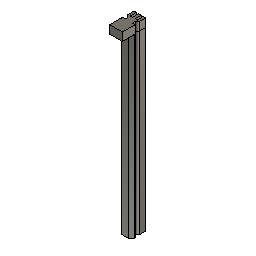
Car Front Cover Slider v1 (Autodesk Fusion 360 design; units mm, degrees)
Autodesk Fusion 360 part; units mm, degrees
note: some values were not read from the file. Set by a fixed rule: which sketch regions a step uses.
sketch "Sketch1" plane through (0, 0, 0) normal (0, 0, 1) x (1, 0, 0)
  line L0 (6.9, 0.5) -> (6.9, -1.8)
  line L1 (6.9, -1.8) -> (4.6, -1.8)
  line L2 (4.6, -1.8) -> (4.6, -2.8)
  line L3 (4.6, -2.8) -> (6.9335, -5.1335)
  line L4 (4.6, -2.8) -> (7.9, -2.8) construction
  line L5 (4.6, -1.8) -> (10.8, -1.8)
  line L6 (6.9, -1.8) -> (13.1, -1.8)
  line L7 (13.1, -1.8) -> (15.4273, -1.8)
  line L8 (15.4273, -1.8) -> (15.4273, -2.8)
  line L9 (15.4273, -2.8) -> (13.0938, -5.1335)
  line L10 (13.0938, -5.1335) -> (6.9335, -5.1335)
  line L11 (15.4273, -1.8) -> (13.1, -1.8)
  line L12 (13.1, -1.8) -> (13.1, 0.5)
  line L13 (6.9, 0.5) -> (4.9, 0.5)
  line L14 (4.9, 0.5) -> (4.9, 7.6)
  line L15 (4.9, 7.6) -> (6.9, 7.6)
  line L16 (6.9, 7.6) -> (6.9, 2.5)
  line L17 (6.9, 2.5) -> (8.875, 2.5)
  line L18 (8.875, 2.5) -> (8.875, 7.6)
  line L19 (8.875, 7.6) -> (10.925, 7.6)
  line L20 (10.925, 7.6) -> (10.925, 2.5)
  line L21 (10.925, 2.5) -> (12.9, 2.5)
  line L22 (12.9, 2.5) -> (12.9, 7.6)
  line L23 (12.9, 7.6) -> (14.9, 7.6)
  line L24 (14.9, 7.6) -> (14.9, 0.5)
  line L25 (14.9, 0.5) -> (13.1, 0.5)
  dimension "d2" = 2.3
  dimension "d3" = 2.3
  dimension "d4" = 1
  dimension "d5" = 45
  dimension "d6" = 3.3
  dimension "d7" = 6.2
  dimension "d11" = 6.2
  dimension "d12" = 135
  dimension "d13" = 3.3
  dimension "d127" = 2.3
  dimension "d128" = 2
  dimension "d129" = 7.1
  dimension "d130" = 2
  dimension "d131" = 5.1
  dimension "d132" = 1.975
  dimension "d133" = 2.05
  dimension "d134" = 1.975
  dimension "d135" = 2
  dimension "d136" = 7.1
  dimension "d143" = 2
  dimension "d144" = 5.1
  constraint perpendicular L0 L1
  constraint perpendicular L1 L2
  constraint horizontal L4
  constraint perpendicular L2 L5
  constraint perpendicular L0 L6
  constraint parallel L6 L7
  constraint perpendicular L7 L8
  constraint perpendicular L11 L12
  constraint perpendicular L0 L13
  constraint perpendicular L13 L14
  constraint perpendicular L14 L15
  constraint perpendicular L15 L16
  constraint perpendicular L16 L17
  constraint perpendicular L17 L18
  constraint perpendicular L18 L19
  constraint perpendicular L19 L20
  constraint perpendicular L20 L21
  constraint perpendicular L21 L22
  constraint perpendicular L22 L23
  constraint perpendicular L21 L24
  constraint perpendicular L12 L25
  measures "d2" distance of L0.start L0.end
  measures "d3" distance of L0.end L1.end
  measures "d4" distance of L1.end L2.end
  measures "d5" angle of L3 L4
  measures "d6" distance of L2.end L3.end
  measures "d7" distance of L1.end L5.end
  measures "d11" distance of L0.end L6.end
  measures "d12" angle of L8 L9
  measures "d13" distance of L8.end L9.end
  measures "d127" distance of L6.end L12.end
  measures "d128" distance of L0.start L13.end
  measures "d129" distance of L13.end L14.end
  measures "d130" distance of L14.end L15.end
  measures "d131" distance of L15.end L16.end
  measures "d132" distance of L16.end L17.end
  measures "d133" distance of L18.end L19.end
  measures "d134" distance of L20.end L21.end
  measures "d135" distance of L22.end L23.end
  measures "d136" distance of L23.end L24.end
  measures "d143" distance of L21 L25
  measures "d144" distance of L19.end L20.end
extrude "Extrude1" add sketch "Sketch1" along normal blind 150 makes body 1
fillet "Fillet5" radius 2 2 edges at (14.9, 0.5, 75) (4.9, 0.5, 75) on bodies 1
sketch "Sketch12" plane through (0, 0, 150) normal (0, 0, 1) x (-1, 0, 0)
  arc A0 (-4.9, -2.5) -> (-6.9, -0.5) centre (-6.9, -2.5) ccw
  line L0 (-6.9, -0.5) -> (-6.9, 1.8)
  line L1 (-6.9, 1.8) -> (-4.6, 1.8)
  line L2 (-4.6, 1.8) -> (-4.6, 2.8)
  line L3 (-4.6, 2.8) -> (-6.9335, 5.1335)
  line L4 (-6.9335, 5.1335) -> (-13.0938, 5.1335)
  line L5 (-13.0938, 5.1335) -> (-15.4273, 2.8)
  line L6 (-15.4273, 2.8) -> (-15.4273, 1.8)
  line L7 (-15.4273, 1.8) -> (-13.1, 1.8)
  line L8 (-13.1, 1.8) -> (-13.1, -0.5)
  arc A1 (-13.1, -0.5) -> (-14.9, -2.49) centre (-12.9, -2.49) ccw
  line L9 (-14.9, -2.49) -> (-14.9, -7.6)
  line L10 (-14.9, -7.6) -> (-12.9, -7.6)
  line L11 (-12.9, -7.6) -> (-12.9, -2.5)
  line L12 (-12.9, -2.5) -> (-10.925, -2.5)
  line L13 (-10.925, -2.5) -> (-10.925, -7.6)
  line L14 (-10.925, -7.6) -> (-8.875, -7.6)
  line L15 (-8.875, -7.6) -> (-8.875, -2.5)
  line L16 (-8.875, -2.5) -> (-6.9, -2.5)
  line L17 (-6.9, -2.5) -> (-6.9, -7.6)
  line L18 (-6.9, -7.6) -> (-4.9, -7.6)
  line L19 (-4.9, -7.6) -> (-4.9, -2.5)
  line L20 (-15.4273, 2.8) -> (-4.6003, 2.8)
  line L21 (-4.6003, 2.8) -> (-4.6003, 12.8)
  line L22 (-4.6003, 12.8) -> (-15.4273, 12.8)
  line L23 (-15.4273, 12.8) -> (-15.4273, 2.8)
  dimension "d145" = 10.827
  dimension "d146" = 10
  constraint horizontal L20
  constraint vertical L21
  constraint horizontal L22
  constraint vertical L23
  constraint coincident L5.end L6.start
  measures "d145" distance of L5.end L20.end
  measures "d146" distance of L5.end L22.end
extrude "Extrude34" add sketch "Sketch12" along normal blind 7 separate body makes body 2
